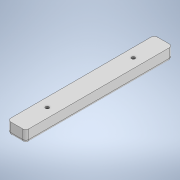
# Autodesk Inventor part: Part12
Saved by Autodesk Inventor 2020 (Build 240168000, 168)
## iProperties
Created: 2019-12-30
Part Number: Part12
Material: Generic
Document SubType Name: Modeling
Designer: tdmp4
Density: 1 g/cm^3
Appearance: Default
Author: tdmp4
Autodesk Inventor part; units mm, degrees
ref_plane "YZ Plane" through (0, 0, 0) normal (1, 0, 0) x (0, 1, 0)
ref_plane "XZ Plane" through (0, 0, 0) normal (0, 1, 0) x (-1, 0, 0)
ref_plane "XY Plane" through (0, 0, 0) normal (0, 0, 1) x (1, 0, 0)
sketch "Sketch1" plane through (0, 0, 0) normal (0, 1, 0) x (-1, 0, 0)
  line L0 (0, 0) -> (19.05, 0)
  line L1 (19.05, 0) -> (19.05, -152.4)
  line L2 (19.05, -152.4) -> (0, -152.4)
  line L3 (0, -152.4) -> (0, 0)
  dimension "d0" = 152.4
  dimension "d1" = 19.05
  constraints: 8 end point, 2 parallel, 1 horizontal, 1 perpendicular
  measures "d0" distance of L0.end L1.end
  measures "d1" distance of L1.end L2.end
extrude "Extrusion1" add sketch "Sketch1" along normal blind 12.7
sketch "Sketch2" plane through (0, 12.7, 0) normal (0, 1, 0) x (1, 0, 0)
  line L0 (-19.05, 0) -> (0, 0) projected
  line L1 (-19.05, 152.4) -> (-19.05, 0) projected
  line L2 (0, 0) -> (-19.05, 152.4)
  line L3 (0, 0) -> (0, 152.4) projected
  line L4 (-19.05, 0) -> (0, 152.4)
  line L5 (-9.525, 76.2) -> (-9.525, 0)
  line L6 (-9.525, 76.2) -> (-9.525, 152.4)
  line L7 (0, 152.4) -> (-19.05, 152.4) projected
  circle A0 centre (-9.525, 31.8589) radius 1.7859
  circle A1 centre (-9.525, 121.157) radius 1.7859
  dimension "d4" = 3.5719
  dimension "d5" = 3.5719
  constraints: 8 end point, 3 midpoint, 2 centre point, 2 point on line
  measures "d4" diameter of A0
  measures "d5" diameter of A1
extrude "Extrusion2" cut sketch "Sketch2" against normal blind 34.925 contours A0 L5 | L5 A0 | A1 L6 | L6 A1
fillet "Fillet1" radius 3.175 8 edges at (0, 6.35, 0) (-19.05, 6.35, 0) (-9.525, 0, 0) (0, 0, -76.2) (0, 6.35, -152.4) (-9.525, 0, -152.4) (-19.05, 6.35, -152.4) (-19.05, 0, -76.2)
body "Solid1"
